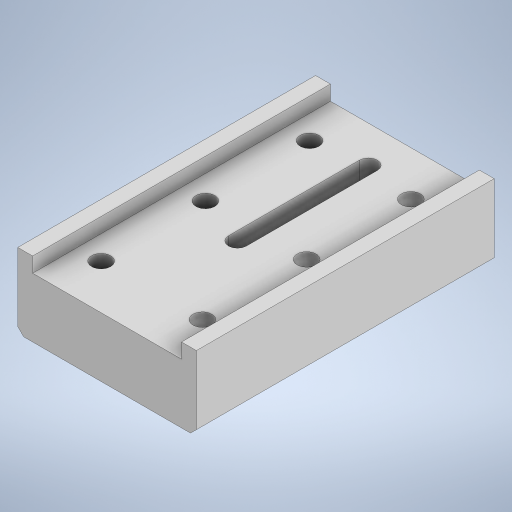
# Autodesk Inventor part: Schneidführungs
Saved by Autodesk Inventor 2023.2 (Build 272271030, 271C)
## iProperties
Created: 2023-02-12
Part Number: Schneidführungs
Material: Generic
Document SubType Name: Modeling
Designer: Ayush
Density: 1 g/cm^3
Appearance: Default
Author: Ayush
Autodesk Inventor part; units mm, degrees
ref_plane "YZ Plane" through (0, 0, 0) normal (1, 0, 0) x (0, 1, 0)
ref_plane "XZ Plane" through (0, 0, 0) normal (0, 1, 0) x (-1, 0, 0)
ref_plane "XY Plane" through (0, 0, 0) normal (0, 0, 1) x (1, 0, 0)
sketch "Sketch1" plane through (0, 0, 0) normal (0, 1, 0) x (-1, 0, 0)
  line L0 (0, 0) -> (-30, 0)
  line L1 (0, 0) -> (30, 0)
  line L2 (30, 0) -> (30, -100)
  line L3 (30, -100) -> (-30, -100)
  line L4 (-30, -100) -> (-30, 0)
  circle A0 centre (17, -85) radius 5.5
  circle A1 centre (17, -50) radius 5.5
  circle A2 centre (17, -15) radius 5.5
  circle A3 centre (-17, -15) radius 5.5
  circle A4 centre (-17, -50) radius 5.5
  circle A5 centre (-17, -85) radius 5.5
  arc A6 (-3, -87.7691) -> (3, -87.7691) centre (0, -87.7691) ccw
  arc A7 (3, -43.7691) -> (-3, -43.7691) centre (0, -43.7691) ccw
  line L5 (3, -87.7691) -> (3, -43.7691)
  line L6 (-3, -87.7691) -> (-3, -43.7691)
  dimension "d0" = 30
  dimension "d1" = 30
  dimension "d2" = 100
  dimension "d3" = 11
  dimension "d4" = 11
  dimension "d5" = 11
  dimension "d6" = 11
  dimension "d7" = 11
  dimension "d8" = 11
  dimension "d9" = 15
  dimension "d10" = 35
  dimension "d11" = 70
  dimension "d12" = 13
  dimension "d13" = 6
  dimension "d14" = 6
  dimension "d15" = 44
  dimension "d16" = 13
  constraints: 14 end point, 8 centre point, 4 point on circle, 3 horizontal alignment, 3 perpendicular, 3 vertical alignment, 2 horizontal, 2 tangent
  measures "d0" distance of L0.start L0.end
  measures "d1" distance of L0.start L1.end
  measures "d2" distance of L1.end L2.end
  measures "d3" diameter of A0
  measures "d4" diameter of A1
  measures "d5" diameter of A2
  measures "d6" diameter of A3
  measures "d7" diameter of A4
  measures "d8" diameter of A5
  measures "d9" distance from line of A3.centre L0
  measures "d10" distance of A4.centre A3.centre
  measures "d11" distance of A5.centre A3.centre
  measures "d12" distance from line of L4 A3.centre
  measures "d13" diameter of A6
  measures "d14" diameter of A7
  measures "d15" distance of A7.centre A6.centre
  measures "d16" distance from line of L2 A0.centre
extrude "Extrusion1" add sketch "Sketch1" along normal blind 6
sketch "Sketch2" plane through (0, 6, 0) normal (0, 1, 0) x (1, 0, 0)
  line L0 (-30, 100) -> (-30, 0) projected
  line L1 (30, 0) -> (30, 100) projected
  line L2 (-30, 100) -> (30, 100)
  line L3 (30, 100) -> (30, 0)
  line L4 (-30, 0) -> (30, 0) projected
  line L5 (-30, 0) -> (-30, 100)
  circle A0 centre (-17, 85) radius 3.2
  circle A1 centre (-17, 15) radius 3.2
  circle A2 centre (17, 15) radius 3.2
  circle A3 centre (17, 50) radius 3.2
  circle A4 centre (17, 85) radius 3.2
  circle A5 centre (-17, 50) radius 3.2
  line L6 (-3, 43.7691) -> (-3, 87.7691) projected
  line L7 (-3, 87.7691) -> (-3, 43.7691)
  line L8 (3, 87.7691) -> (3, 43.7691) projected
  line L9 (3, 87.7691) -> (3, 43.7691)
  arc A6 (3, 87.7691) -> (-3, 87.7691) centre (0, 87.7691) ccw
  arc A7 (-3, 43.7691) -> (3, 43.7691) centre (0, 43.7691) ccw projected
  arc A8 (-3, 43.7691) -> (3, 43.7691) centre (0, 43.7691) ccw
  point P0 (0, 0)
  dimension "d19" = 6.4
  dimension "d21" = 6.4
  dimension "d22" = 6.4
  dimension "d23" = 6.4
  dimension "d24" = 6.4
  dimension "d25" = 15
  dimension "d26" = 35
  dimension "d27" = 70
  dimension "d28" = 13
  dimension "d29" = 13
  dimension "d30" = 6.4
  dimension "d31" = 6
  constraints: 10 end point, 8 centre point, 4 collinear, 4 point on circle, 3 horizontal alignment, 2 vertical alignment, 1 horizontal, 1 tangent
  measures "d19" diameter of A0
  measures "d21" diameter of A1
  measures "d22" diameter of A2
  measures "d23" diameter of A3
  measures "d24" diameter of A4
  measures "d25" distance from line of A2.centre L4
  measures "d26" distance of A3.centre A2.centre
  measures "d27" distance of A4.centre A2.centre
  measures "d28" distance from line of A2.centre L1
  measures "d29" distance from line of A1.centre L0
  measures "d30" diameter of A5
  measures "d31" diameter of A6
extrude "Extrusion2" add sketch "Sketch2" along normal blind 14
sketch "Sketch4" plane through (30, 20, -100) normal (0, 0, -1) x (-1, 0, 0)
  circle A0 centre (20, -10) radius 4
  circle A1 centre (40, -10) radius 4
  line L0 (0, 0) -> (60, 0) projected
  line L1 (0, -20) -> (0, 0) projected
  line L2 (60, -20) -> (60, 0) projected
  point P0 (30, -20)
  point P1 (0, -25)
  point P2 (60, -25)
  dimension "d43" = 8
  dimension "d44" = 8
  dimension "d45" = 10
  dimension "d46" = 20
  dimension "d47" = 20
  constraints: 2 centre point, 1 horizontal alignment
  measures "d43" diameter of A0
  measures "d44" diameter of A1
  measures "d45" distance from line of A1.centre L0
  measures "d46" distance from line of A0.centre L1
  measures "d47" distance from line of A1.centre L2
hole "Hole1" at (-10, 10, -100) at (10, 10, -100) direction (0, 0, 1) diameter 8 depth 12 tip angle 118
sketch "Sketch5" plane through (0, 20, 0) normal (0, 1, 0) x (1, 0, 0)
  line L0 (30, 100) -> (-30, 100) projected
  line L1 (30, 0) -> (30, 100) projected
  line L2 (30, 100) -> (30, 0)
  line L3 (30, 0) -> (25, 0)
  line L4 (-30, 0) -> (30, 0) projected
  line L5 (25, 0) -> (25, 100)
  line L6 (25, 100) -> (30, 100)
  line L7 (-30, 100) -> (-30, 0) projected
  line L8 (-30, 100) -> (-30, 0)
  line L9 (-30, 0) -> (-25, 0)
  line L10 (-25, 0) -> (-25, 100)
  line L11 (-30, 100) -> (-25, 100)
  point P0 (0, 0)
  dimension "d55" = 100
  dimension "d56" = 5
  dimension "d57" = 100
  dimension "d58" = 5
  constraints: 16 end point, 3 collinear, 3 perpendicular, 3 point on line
  measures "d55" distance of L0.start L1.start
  measures "d56" distance of L1.start L3.end
  measures "d57" distance of L0.end L4.start
  measures "d58" distance of L4.start L9.end
extrude "Extrusion4" add sketch "Sketch5" along normal blind 5 contours L1 L3 L5 L0 | L10 L4 L7 L0
chamfer "Chamfer1" distance 2 angle 45 1 edges at (-30, 0, -50) measured on face at (27.5, 0, -50)
chamfer "Chamfer2" distance 2 angle 45 1 edges at (30, 0, -50) measured on face at (27.5, 0, -50)
body "Solid1"
